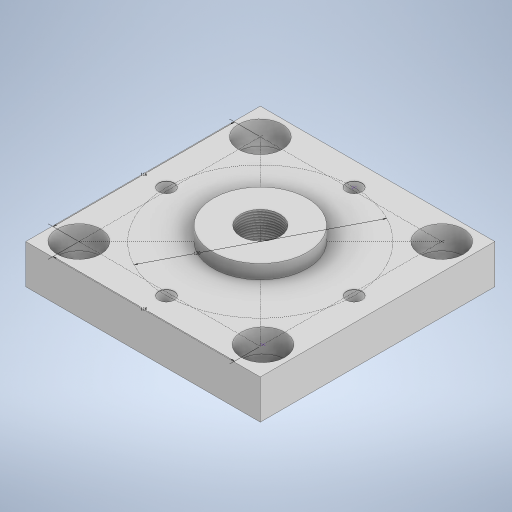
# Autodesk Inventor part: BasePlate
Saved by Autodesk Inventor 2024 (Build 280153000, 153)
## iProperties
Created: 2023-11-09
Part Number: BasePlate
Material: Generic
Document SubType Name: Modeling
Designer: Admin
Density: 1 g/cm^3
Appearance: Default
Author: Admin
Autodesk Inventor part; units mm, degrees
ref_plane "YZ Plane" through (0, 0, 0) normal (1, 0, 0) x (0, 1, 0)
ref_plane "XZ Plane" through (0, 0, 0) normal (0, 1, 0) x (-1, 0, 0)
ref_plane "XY Plane" through (0, 0, 0) normal (0, 0, 1) x (1, 0, 0)
sketch "Sketch1" plane through (0, 0, 0) normal (0, 1, 0) x (-1, 0, 0)
  line L0 (-75, -75) -> (75, -75)
  line L1 (75, -75) -> (75, 75)
  line L2 (75, 75) -> (-75, 75)
  line L3 (-75, 75) -> (-75, -75)
  line L4 (-75, -75) -> (75, 75) construction
  line L5 (75, -75) -> (-75, 75) construction
  point P0 (0, 0)
  dimension "d0" = 150
  dimension "d1" = 150
  constraints: 12 end point, 2 midpoint, 2 parallel, 1 horizontal, 1 perpendicular
  measures "d0" distance of L2.end L1.end
  measures "d1" distance of L1.end L0.end
extrude "Extrusion1" add sketch "Sketch1" along normal blind 25
sketch "Sketch2" plane through (0, 25, 0) normal (0, 1, 0) x (1, 0, 0)
  circle A0 centre (0, 0) radius 30
  dimension "d4" = 60
  constraints: 1 centre point, 1 coincident
  measures "d4" diameter of A0
sketch "Sketch3" plane through (0, 25, 0) normal (0, 1, 0) x (1, 0, 0)
  line L0 (58, 58) -> (-58, 58) construction
  line L1 (-58, 58) -> (-58, -58) construction
  line L2 (-58, -58) -> (58, -58) construction
  line L3 (58, -58) -> (58, 58) construction
  line L4 (58, 58) -> (-58, -58) construction
  line L5 (-58, 58) -> (58, -58) construction
  circle A0 centre (0, 0) radius 60 construction
  point P0 (58, -56.2544)
  point P1 (0, 60)
  dimension "d7" = 120
  dimension "d5" = 116
  dimension "d6" = 116
  constraints: 12 end point, 4 coincident, 2 midpoint, 2 parallel, 1 horizontal, 1 perpendicular, 1 point on line, 1 vertical alignment, 2 other
  measures "d5" distance of L2.end L1.end
  measures "d6" distance of L1.end L0.end
extrude "Extrusion2" add sketch "Sketch2" along normal blind 9
hole "Hole1" at (-58, 25, -58) at (58, 25, -58) at (58, 25, 56.2544) at (-58, 25, 58) direction (0, -1, 0) diameter 28 depth 15 tip angle 100
hole "Hole2" at (0, 25, -60) direction (0, -1, 0) diameter 10 depth 0.2 tip angle 90
pattern_circular "Circular Pattern1" count 4 over 360 about axis through (0, 25, 0) along (0, 1, 0) of "Hole2"
sketch "Sketch4" plane through (0, 0, 0) normal (0, -1, 0) x (1, 0, 0)
  circle A0 centre (58, -58) radius 2.0825 projected
  circle A1 centre (-58, -58) radius 2.0825 projected
  circle A2 centre (-58, 58) radius 2.0825 projected
  circle A3 centre (58, 56.2544) radius 2.0825 projected
  point P0 (0, 0)
  constraints: 4 coincident
hole "Hole3" at (58, 0, -58) at (-58, 0, -58) at (-58, 0, 58) at (58, 0, 56.2544) direction (0, 1, 0) diameter 17 end through all
sketch "Sketch5" plane through (0, 34, 0) normal (0, 1, 0) x (1, 0, 0)
  circle A0 centre (0, 0) radius 30 construction
hole "Hole5" at (0, 34, 0) direction (0, -1, 0) diameter 25 end through all
thread "Thread1" size "M25x1.5" class "6H" standard "ANSI Metric M Profile" length 30
body "Solid1"
